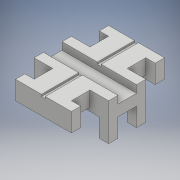
# Autodesk Inventor part: CableGuide
Saved by Autodesk Inventor 2018 (Build 220112000, 112)
## iProperties
Created: 2018-05-09
Part Number: CableGuide
Material: Generic
Document SubType Name: Modeling
Designer: s4321966
Density: 1 g/cm^3
Appearance: Default
Mass: 1.69 g
Surface Area: 15.98 cm^2
Volume: 1.69 cm^3
Author: s4321966
Autodesk Inventor part; units mm, degrees
ref_plane "YZ Plane" through (0, 0, 0) normal (1, 0, 0) x (0, 1, 0)
ref_plane "XZ Plane" through (0, 0, 0) normal (0, 1, 0) x (-1, 0, 0)
ref_plane "XY Plane" through (0, 0, 0) normal (0, 0, 1) x (1, 0, 0)
sketch "Sketch1" plane through (0, 0, 0) normal (0, 0, 1) x (1, 0, 0)
  line L0 (0, 0) -> (20, 0)
  line L1 (20, 0) -> (20, -2.7984)
  line L2 (0, -2.7984) -> (0, 0)
  line L3 (0, 0) -> (20, 0)
  line L4 (20, 0) -> (20, -50)
  line L5 (20, -50) -> (0, -50)
  line L6 (0, -50) -> (0, 0)
  line L7 (0, 0) -> (5, 0)
  line L8 (0, -5) -> (0, 0)
  circle A0 centre (5, -5) radius 1.651
  line L9 (20, 0) -> (15, 0)
  line L10 (15, -5) -> (20, -5)
  line L11 (20, -5) -> (20, 0)
  circle A1 centre (15, -5) radius 1.651
  dimension "d1" = 20
  dimension "d2" = 50
  dimension "d6" = 5
  dimension "d7" = 5
  dimension "d9" = 3.302
  constraints: 24 end point, 4 horizontal, 4 parallel, 2 centre point, 2 perpendicular
  measures "d1" distance of L4.end L5.end
  measures "d2" distance of L3.end L4.end
  measures "d6" distance of L10.end L10.start
  measures "d7" distance of L10.start L9.end
  measures "d9" diameter of A1
extrude "Extrusion1" add sketch "Sketch1" along normal blind 5
sketch "Sketch2" plane through (0, 0, 5) normal (0, 0, 1) x (1, 0, 0)
  line L0 (20, 0) -> (0, 0) projected
  line L1 (10, 0) -> (5, 0)
  line L2 (5, 0) -> (5, 5)
  line L3 (5, 5) -> (10, 5)
  line L4 (10, 5) -> (10, 0)
  line L5 (10, 5) -> (2.5, 5)
  line L6 (2.5, 5) -> (2.5, 7.5)
  line L7 (2.5, 7.5) -> (10, 7.5)
  line L8 (10, 7.5) -> (10, 5)
  line L9 (2.5, 7.5) -> (17.5, 7.5)
  line L10 (17.5, 7.5) -> (17.5, 5)
  line L11 (17.5, 5) -> (2.5, 5)
  line L12 (2.5, 5) -> (2.5, 7.5)
  line L13 (10, 5) -> (15, 5)
  line L14 (15, 5) -> (15, 0)
  line L15 (15, 0) -> (10, 0)
  line L16 (10, 0) -> (10, 5)
  dimension "d12" = 5
  dimension "d13" = 5
  dimension "d14" = 7.5
  dimension "d15" = 2.5
  dimension "d16" = 15
  dimension "d17" = 2.5
  dimension "d18" = 5
  dimension "d19" = 5
  constraints: 32 end point, 8 parallel, 4 horizontal, 4 perpendicular, 1 midpoint
  measures "d12" distance of L2.end L3.end
  measures "d13" distance of L1.end L2.end
  measures "d14" distance of L6.end L7.end
  measures "d15" distance of L5.end L6.end
  measures "d16" distance of L10.end L11.end
  measures "d17" distance of L9.end L10.end
  measures "d18" distance of L14.end L15.end
  measures "d19" distance of L13.end L14.end
extrude "Extrusion2" add sketch "Sketch2" against normal blind 5
sketch "Sketch3" plane through (0, 0, 0) normal (0, 0, -1) x (-1, 0, 0)
  line L0 (-5, 0) -> (-5, 5) projected
  line L1 (-5, 0) -> (-15, 0)
  line L2 (-15, 0) -> (-15, 5)
  line L3 (-15, 5) -> (-5, 5)
  line L4 (-5, 5) -> (-5, 0)
  point P0 (0, 0)
  constraints: 8 end point, 2 parallel, 1 horizontal, 1 perpendicular
extrude "Extrusion3" cut sketch "Sketch3" against normal blind 1
sketch "Sketch4" plane through (0, 0, 0) normal (0, 0, -1) x (-1, 0, 0)
  line L0 (-5, 0) -> (0, 0) projected
  line L1 (-20, -50) -> (0, -50) projected
  line L2 (0, 0) -> (-20, 0)
  line L3 (-20, 0) -> (-20, -50)
  line L4 (-20, -50) -> (0, -50)
  line L5 (0, -50) -> (0, 0)
  line L6 (0, -50) -> (-5, -50)
  line L7 (-5, -50) -> (-5, -30)
  line L8 (-5, -30) -> (0, -30)
  line L9 (0, -30) -> (0, -50)
  line L10 (0, -50) -> (0, 0) projected
  line L11 (0, -50) -> (-5, -50)
  line L12 (-5, -50) -> (-5, -30)
  line L13 (-5, -30) -> (0, -30)
  line L14 (0, -30) -> (0, -50)
  line L15 (0, -50) -> (-20, -50)
  line L16 (-20, -50) -> (-20, -45)
  line L17 (-20, -45) -> (0, -45)
  line L18 (0, -45) -> (0, -50)
  dimension "d28" = 5
  dimension "d29" = 20
  dimension "d30" = 5
  dimension "d31" = 20
  dimension "d32" = 20
  dimension "d33" = 5
  constraints: 32 end point, 8 parallel, 4 horizontal, 4 perpendicular
  measures "d28" distance of L7.end L8.end
  measures "d29" distance of L6.end L7.end
  measures "d30" distance of L7.end L13.end
  measures "d31" distance of L11.end L7.end
  measures "d32" distance of L16.end L17.end
  measures "d33" distance of L15.end L16.end
extrude "Extrusion4" add sketch "Sketch4" along normal blind 15 contours L17 L7 L1 L3 | L5 L1 L7 L17
sketch "Sketch5" plane through (0, 0, 5) normal (0, 0, 1) x (1, 0, 0)
  line L0 (20, -50) -> (20, 0) projected
  line L1 (20, 0) -> (0, 0)
  line L2 (0, 0) -> (0, -50)
  line L3 (0, -50) -> (20, -50)
  line L4 (20, -50) -> (20, 0)
  line L5 (10, -50) -> (15, -50)
  line L6 (15, -50) -> (15, -55)
  line L7 (15, -55) -> (10, -55)
  line L8 (10, -55) -> (10, -50)
  line L9 (15, -55) -> (5, -55)
  line L10 (5, -55) -> (5, -50)
  line L11 (5, -50) -> (15, -50)
  line L12 (15, -50) -> (15, -55)
  line L13 (10, -55) -> (17.5, -55)
  line L14 (17.5, -55) -> (17.5, -57.5)
  line L15 (17.5, -57.5) -> (10, -57.5)
  line L16 (10, -57.5) -> (10, -55)
  line L17 (17.5, -57.5) -> (2.5, -57.5)
  line L18 (2.5, -57.5) -> (2.5, -55)
  line L19 (2.5, -55) -> (17.5, -55)
  line L20 (17.5, -55) -> (17.5, -57.5)
  dimension "d36" = 5
  dimension "d37" = 5
  dimension "d38" = 10
  dimension "d39" = 5
  dimension "d40" = 7.5
  dimension "d41" = 2.5
  dimension "d42" = 15
  dimension "d43" = 2.5
  constraints: 40 end point, 10 parallel, 5 horizontal, 5 perpendicular, 1 midpoint
  measures "d36" distance of L6.end L7.end
  measures "d37" distance of L5.end L6.end
  measures "d38" distance of L10.end L11.end
  measures "d39" distance of L9.end L10.end
  measures "d40" distance of L14.end L15.end
  measures "d41" distance of L13.end L14.end
  measures "d42" distance of L18.end L19.end
  measures "d43" distance of L17.end L18.end
extrude "Extrusion5" add sketch "Sketch5" against normal blind 5 contours L6 L7 L8 L3 | L8 L9 L10 L3 | L13 L14 L15 L16 L7 | L16 L17 L18 L19 L9
sketch "Sketch6" plane through (0, 0, 0) normal (0, 0, -1) x (-1, 0, 0)
  line L0 (-5, -55) -> (-5, -50) projected
  line L1 (-15, -50) -> (-5, -50) projected
  line L2 (-5, -55) -> (-15, -55)
  line L3 (-15, -55) -> (-15, -50)
  line L4 (-15, -50) -> (-5, -50)
  line L5 (-5, -50) -> (-5, -55)
  point P0 (0, 0)
  constraints: 8 end point, 2 parallel, 1 horizontal, 1 perpendicular
extrude "Extrusion6" cut sketch "Sketch6" against normal blind 1
sketch "Sketch8" plane through (0, -45, 0) normal (0, 1, 0) x (1, 0, 0)
  line L0 (0, 15) -> (20, 15) projected
  line L1 (0, 15) -> (20, 15)
  line L2 (20, 15) -> (20, 0)
  line L3 (20, 0) -> (0, 0)
  line L4 (0, 0) -> (0, 15)
  line L5 (0, 0) -> (0, 15) projected
  line L6 (0, 7.5) -> (20, 7.5)
  line L7 (20, 0) -> (20, 15) projected
  line L8 (20, 0) -> (0, 15)
  line L9 (20, 15) -> (0, 0)
  line L10 (10, 7.5) -> (10, 15)
  line L11 (10, 7.5) -> (10, 0)
  line L12 (10, 7.5) -> (0, 0)
  line L13 (10, 7.5) -> (20, 0)
  line L14 (10, 7.5) -> (0, 15)
  line L15 (10, 7.5) -> (20, 15)
  circle A0 centre (5, 3.75) radius 1.651
  circle A1 centre (15, 3.75) radius 1.651
  circle A2 centre (15, 11.25) radius 1.651
  circle A3 centre (5, 11.25) radius 1.651
  dimension "d48" = 3.302
  dimension "d49" = 3.302
  dimension "d50" = 3.302
  dimension "d51" = 3.302
  constraints: 26 end point, 9 midpoint, 4 centre point, 4 collinear, 2 parallel, 1 horizontal, 1 perpendicular
  measures "d48" diameter of A0
  measures "d49" diameter of A1
  measures "d50" diameter of A2
  measures "d51" diameter of A3
extrude "Extrusion7" cut sketch "Sketch8" against normal blind 5 contours A3 L8 | L8 A3 | A2 L9 | L9 A2 | A1 L8 | L8 A1 | A0 L9 | L9 A0
sketch "Sketch9" plane through (0, 0, 0) normal (0, 0, -1) x (-1, 0, 0)
  line L0 (6.3074, -39.8098) -> (-37.7059, -39.8098)
  line L1 (-37.7059, -39.8098) -> (-37.7059, -53.6211)
  line L2 (-37.7059, -53.6211) -> (6.3074, -53.6211)
  line L3 (6.3074, -53.6211) -> (6.3074, -39.8098)
  point P0 (0, 0)
  constraints: 8 end point, 2 parallel, 1 horizontal, 1 perpendicular
extrude "Extrusion8" cut sketch "Sketch9" along normal blind 100
sketch "Sketch10" plane through (0, 0, 0) normal (0, 0, -1) x (-1, 0, 0)
  line L0 (0, 0) -> (0, -50) projected
  line L1 (-20, -50) -> (-20, 0) projected
  line L2 (0, -50) -> (-20, -50)
  line L3 (-20, -50) -> (-20, -40)
  line L4 (-20, -40) -> (0, -40)
  line L5 (0, -40) -> (0, -50)
  line L6 (-20, -40) -> (0, -40)
  line L7 (0, -40) -> (0, 19.6469)
  line L8 (0, 19.6469) -> (-20, 19.6469)
  line L9 (-20, 19.6469) -> (-20, -40)
  dimension "d56" = 10
  constraints: 16 end point, 4 parallel, 2 horizontal, 2 perpendicular, 2 point on line
  measures "d56" distance of L2.end L3.end
extrude "Extrusion9" cut sketch "Sketch10" against normal blind 100 contours L0 L4 L1 L9 L8 L7
sketch "Sketch11" plane through (0, 0, 5) normal (0, 0, 1) x (1, 0, 0)
  line L0 (0, -40) -> (20, -40) projected
  line L1 (10, -40) -> (15, -40)
  line L2 (15, -40) -> (15, -35)
  line L3 (15, -35) -> (10, -35)
  line L4 (10, -35) -> (10, -40)
  line L5 (10, -35) -> (17.5, -35)
  line L6 (17.5, -35) -> (17.5, -32.5)
  line L7 (17.5, -32.5) -> (10, -32.5)
  line L8 (10, -32.5) -> (10, -35)
  line L9 (17.5, -32.5) -> (2.5, -32.5)
  line L10 (2.5, -32.5) -> (2.5, -35)
  line L11 (2.5, -35) -> (17.5, -35)
  line L12 (17.5, -35) -> (17.5, -32.5)
  line L13 (10, -35) -> (5, -35)
  line L14 (5, -35) -> (5, -40)
  line L15 (5, -40) -> (10, -40)
  line L16 (10, -40) -> (10, -35)
  point P0 (0, 0)
  dimension "d59" = 5
  dimension "d60" = 5
  dimension "d61" = 7.5
  dimension "d62" = 2.5
  dimension "d63" = 15
  dimension "d64" = 2.5
  dimension "d65" = 5
  dimension "d66" = 5
  constraints: 32 end point, 8 parallel, 4 horizontal, 4 perpendicular, 1 midpoint
  measures "d59" distance of L3.end L2.end
  measures "d60" distance of L2.end L1.end
  measures "d61" distance of L7.end L6.end
  measures "d62" distance of L6.end L5.end
  measures "d63" distance of L11.end L10.end
  measures "d64" distance of L10.end L9.end
  measures "d65" distance of L15.end L14.end
  measures "d66" distance of L14.end L13.end
extrude "Extrusion10" add sketch "Sketch11" against normal blind 5
sketch "Sketch12" plane through (0, 0, 0) normal (0, 0, -1) x (-1, 0, 0)
  line L0 (-15, -35) -> (-15, -40) projected
  line L1 (-5, -40) -> (0, -40) projected
  line L2 (-15, -35) -> (-5, -35)
  line L3 (-5, -35) -> (-5, -40)
  line L4 (-5, -40) -> (-15, -40)
  line L5 (-15, -40) -> (-15, -35)
  point P0 (0, 0)
  constraints: 8 end point, 2 parallel, 1 horizontal, 1 perpendicular
extrude "Extrusion11" cut sketch "Sketch12" against normal blind 1
sketch "Sketch13" plane through (20, -50, 5) normal (1, 0, 0) x (0, 0, -1)
  line L0 (5, 10) -> (0, 10) projected
  line L1 (0, 0) -> (5, 0) projected
  line L2 (5, 10) -> (0, 10)
  line L3 (0, 10) -> (0, 0)
  line L4 (0, 0) -> (5, 0)
  line L5 (5, 0) -> (5, 10)
  line L6 (0, 0) -> (0, 10) projected
  line L7 (0, 5) -> (2, 5)
  line L8 (2, 5) -> (2, 2.5)
  line L9 (2, 2.5) -> (0, 2.5)
  line L10 (0, 2.5) -> (0, 5)
  line L11 (2, 2.5) -> (0, 2.5)
  line L12 (0, 2.5) -> (0, 7.5)
  line L13 (0, 7.5) -> (2, 7.5)
  line L14 (2, 7.5) -> (2, 2.5)
  point P0 (5, 50)
  dimension "d71" = 2
  dimension "d72" = 2.5
  dimension "d73" = 5
  constraints: 24 end point, 6 parallel, 3 horizontal, 3 perpendicular, 1 midpoint, 1 point on line
  measures "d71" distance of L8.end L9.end
  measures "d72" distance of L7.end L8.end
  measures "d73" distance of L11.end L12.end
extrude "Extrusion12" cut sketch "Sketch13" against normal blind 20 contours L13 L14 L7 L3 | L7 L8 L9 L3
sketch "Sketch14" plane through (0, 0, 0) normal (0, 0, -1) x (-1, 0, 0)
  line L0 (-20, -40) -> (-15, -40) projected
  line L1 (-20, -40) -> (-17.5, -40)
  line L2 (-17.5, -40) -> (-17.5, -42.5)
  line L3 (-17.5, -42.5) -> (-20, -42.5)
  line L4 (-20, -42.5) -> (-20, -40)
  line L5 (-15, -50) -> (-20, -50) projected
  line L6 (-20, -50) -> (-17.5, -50)
  line L7 (-17.5, -50) -> (-17.5, -47.5)
  line L8 (-17.5, -47.5) -> (-20, -47.5)
  line L9 (-20, -47.5) -> (-20, -50)
  line L10 (0, -50) -> (0, -40) projected
  line L11 (0, -40) -> (-2.5, -40)
  line L12 (-2.5, -40) -> (-2.5, -42.5)
  line L13 (-2.5, -42.5) -> (0, -42.5)
  line L14 (0, -42.5) -> (0, -40)
  line L15 (0, -50) -> (-2.5, -50)
  line L16 (-2.5, -50) -> (-2.5, -47.5)
  line L17 (-2.5, -47.5) -> (0, -47.5)
  line L18 (0, -47.5) -> (0, -50)
  point P0 (0, 0)
  dimension "d76" = 2.5
  dimension "d77" = 2.5
  dimension "d78" = 2.5
  dimension "d79" = 2.5
  dimension "d80" = 2.5
  dimension "d81" = 2.5
  dimension "d82" = 2.5
  dimension "d83" = 2.5
  constraints: 32 end point, 8 parallel, 4 horizontal, 4 perpendicular
  measures "d76" distance of L2.end L3.end
  measures "d77" distance of L1.end L2.end
  measures "d78" distance of L8.end L7.end
  measures "d79" distance of L7.end L6.end
  measures "d80" distance of L13.end L12.end
  measures "d81" distance of L12.end L11.end
  measures "d82" distance of L16.end L17.end
  measures "d83" distance of L15.end L16.end
extrude "Extrusion13" add sketch "Sketch14" along normal blind 5
sketch "Sketch15" plane through (2.5, -57.5, 5) normal (0, -1, 0) x (1, 0, 0)
  line L0 (17.5, 0) -> (-2.5, 0) projected
  line L1 (7.5, 0) -> (7, 0)
  line L2 (7, 0) -> (7, -0.5)
  line L3 (7, -0.5) -> (7.5, -0.5)
  line L4 (7.5, -0.5) -> (7.5, 0)
  line L5 (7, 0) -> (8, 0)
  line L6 (8, 0) -> (8, -0.5)
  line L7 (8, -0.5) -> (7, -0.5)
  line L8 (7, -0.5) -> (7, 0)
  point P0 (-2.5, -5)
  dimension "d86" = 0.5
  dimension "d87" = 0.5
  dimension "d88" = 1
  dimension "d89" = 0.5
  constraints: 16 end point, 4 parallel, 2 horizontal, 2 perpendicular, 1 midpoint
  measures "d86" distance of L3.end L2.end
  measures "d87" distance of L2.end L1.end
  measures "d88" distance of L6.end L7.end
  measures "d89" distance of L5.end L6.end
extrude "Extrusion14" cut sketch "Sketch15" against normal blind 500
body "Solid1"
